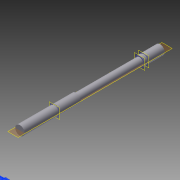
# Autodesk Inventor part: ShaftStraight
Saved by Autodesk Inventor 2012 (Build 160160000, 160)
## iProperties
Created: 2012-02-22
Part Number: ShaftStraight
Material: Aluminum-6061
Document SubType Name: Modeling
Designer: admin
Density: 2.71 g/cm^3
Mass: 6.8205 g
Surface Area: 18.3104 cm^2
Volume: 2.51679 cm^3
Author: admin
Autodesk Inventor part; units mm, degrees
ref_plane "YZ Plane" through (0, 0, 0) normal (1, 0, 0) x (0, 1, 0)
ref_plane "XY Plane" through (0, 0, 0) normal (0, 0, 1) x (1, 0, 0)
sketch "Sketch1" plane through (0, 0, 0) normal (0, 0, 1) x (1, 0, 0)
  circle A0 centre (0, 0) radius 3.175
  dimension "d0" = 6.35
  constraints: 1 centre point, 1 coincident
  measures "d0" diameter of A0
extrude "Extrusion1" add sketch "Sketch1" against normal blind 95.25
ref_plane "Work Plane5" through (0, 0, -81.28) normal (0, 0, -1) x (-1, 0, 0)
sketch "Sketch6" plane through (0, 0, -81.28) normal (0, 0, -1) x (-1, 0, 0)
  circle A0 centre (0, 0) radius 2.54
  circle A1 centre (0, 0) radius 3.175
  dimension "d11" = 5.08
  dimension "d12" = 6.35
  constraints: 2 centre point, 2 coincident
  measures "d11" diameter of A0
  measures "d12" diameter of A1
extrude "Extrusion4" cut sketch "Sketch6" against normal blind 43.18
ref_plane "Work Plane6" through (0, 0, -84.074) normal (0, 0, -1) x (-1, 0, 0)
sketch "Sketch7" plane through (0, 0, -84.074) normal (0, 0, -1) x (-1, 0, 0)
  circle A0 centre (0, 0) radius 3.175
  circle A1 centre (0, 0) radius 2.921
  dimension "d16" = 6.35
  dimension "d17" = 5.842
  constraints: 2 centre point, 2 coincident
  measures "d16" diameter of A0
  measures "d17" diameter of A1
extrude "Extrusion5" cut sketch "Sketch7" against normal blind 0.762
ref_plane "Work Plane7" through (0, 0, -23.368) normal (0, 0, -1) x (-1, 0, 0)
sketch "Sketch8" plane through (0, 0, -23.368) normal (0, 0, -1) x (-1, 0, 0)
  circle A0 centre (0, 0) radius 3.175
  circle A1 centre (0, 0) radius 2.921
  dimension "d21" = 6.35
  dimension "d22" = 5.842
  constraints: 2 centre point, 2 coincident
  measures "d21" diameter of A0
  measures "d22" diameter of A1
extrude "Extrusion6" cut sketch "Sketch8" along normal blind 0.762
body "Solid1"
